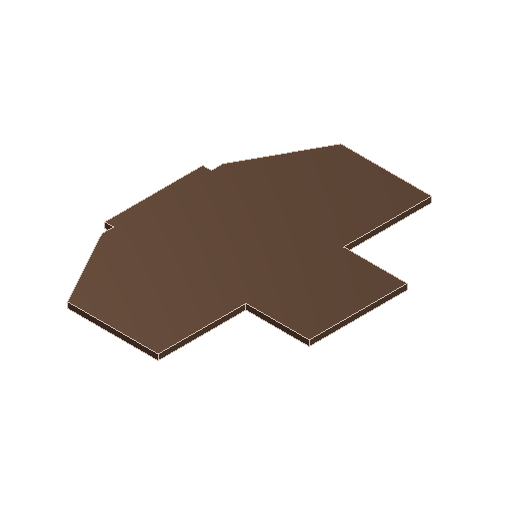
# Autodesk Inventor part: cover
Saved by Autodesk Inventor 2025.2 (Build 292293000, 293)
## iProperties
Created: 2025-03-28
Part Number: cover
Material: 청동, 주조
Document SubType Name: Modeling
Designer: jbhma
Density: 8.87 g/cm^3
Appearance: 청동 - 새틴
Author: jbhma
Autodesk Inventor part; units mm, degrees
ref_plane "YZ Plane" through (0, 0, 0) normal (1, 0, 0) x (0, 1, 0)
ref_plane "XZ Plane" through (0, 0, 0) normal (0, 1, 0) x (-1, 0, 0)
ref_plane "XY Plane" through (0, 0, 0) normal (0, 0, 1) x (1, 0, 0)
sketch "스케치1" plane through (0, 0, 0) normal (0, 1, 0) x (-1, 0, 0)
  line L0 (0, 0) -> (-315, 0)
  line L1 (-315, 0) -> (-315, -950)
  line L2 (-315, -950) -> (0, -950)
  line L3 (0, -950) -> (0, 0)
  line L4 (-315, -645) -> (-315, -475)
  line L5 (-315, -475) -> (-535, -475)
  line L6 (-535, -475) -> (-535, -645)
  line L7 (-535, -645) -> (-315, -645)
  line L8 (-315, -645) -> (-315, -475)
  line L9 (-315, -475) -> (-535, -475)
  line L10 (-315, -305) -> (-315, -475)
  line L11 (-315, -475) -> (-535, -475)
  line L12 (-535, -475) -> (-535, -305)
  line L13 (-535, -305) -> (-315, -305)
  line L14 (-315, -305) -> (-315, -475)
  line L15 (0, -305) -> (0, 0)
  line L16 (0, -645) -> (0, -950)
  line L17 (0, 0) -> (175, 0)
  line L18 (175, 0) -> (175, -950)
  line L19 (175, -950) -> (0, -950)
  line L20 (0, -950) -> (0, 0)
  line L21 (175, 0) -> (145, 0)
  line L22 (145, 0) -> (145, -950)
  line L23 (145, -950) -> (175, -950)
  line L24 (175, -950) -> (175, 0)
  line L25 (175, -475) -> (145, -475)
  line L26 (145, -475) -> (145, -645)
  line L27 (145, -645) -> (175, -645)
  line L28 (175, -645) -> (175, -475)
  line L29 (175, -475) -> (145, -475)
  line L30 (145, -475) -> (145, -305)
  line L31 (145, -305) -> (175, -305)
  line L32 (175, -305) -> (175, -475)
  line L33 (145, -645) -> (-315, -645)
  line L34 (-315, -645) -> (-315, -685)
  line L35 (-315, -685) -> (145, -685)
  line L36 (145, -685) -> (145, -645)
  line L37 (145, -305) -> (-315, -305)
  line L38 (-315, -305) -> (-315, -265)
  line L39 (-315, -265) -> (145, -265)
  line L40 (145, -265) -> (145, -305)
  line L41 (0, 0) -> (145, -265)
  line L42 (145, -685) -> (0, -950)
  dimension "d0" = 315
  dimension "d1" = 950
  dimension "d3" = 220
  dimension "d4" = 170
  dimension "d5" = 220
  dimension "d6" = 170
  dimension "d7" = 175
  dimension "d8" = 30
  dimension "d9" = 460
  dimension "d10" = 40
  dimension "d11" = 460
  dimension "d12" = 40
  constraints: 86 end point, 18 parallel, 10 horizontal, 9 perpendicular, 3 point on line, 2 midpoint
  measures "d0" distance of L2.end L1.end
  measures "d1" distance of L1.end L0.end
  measures "d3" distance of L7.end L6.end
  measures "d4" distance of L6.end L5.end
  measures "d5" distance of L12.end L13.end
  measures "d6" distance of L11.end L12.end
  measures "d7" distance of L18.end L19.end
  measures "d8" distance of L23.end L22.end
  measures "d9" distance of L35.end L34.end
  measures "d10" distance of L34.end L33.end
  measures "d11" distance of L38.end L39.end
  measures "d12" distance of L37.end L38.end
extrude "돌출1" add sketch "스케치1" along normal blind 20 contours L3 L39 L1 L0 | L41 L39 L3 | L39 L22 L37 L3 | L3 L37 L1 L39 | L37 L22 L33 L3 | L3 L33 L1 L37 | L31 L18 L25 L22 | L1 L5 L12 L13 | L33 L22 L35 L3 | L3 L35 L1 L33 | L25 L18 L27 L22 | L1 L7 L6 L5 | L35 L42 L3 | L3 L2 L1 L35
